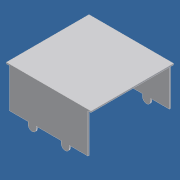
# Autodesk Inventor part: M20_ang_t_shorud2830TX-switch
Saved by Autodesk Inventor 2014 (Build 180170000, 170)
## iProperties
Category: PARTsolutions
Created: 2013-12-29
Part Number: M20_ang_t_shorud2830TX-switch
Catalog Web Link: www.cadenas.de
Description: Angle Mount Miniature Rockers- Switch - Shroud - Series M - Miniature Toggle
Document SubType Name: Modeling
Designer: PARTsolutions
Material: Generic
Density: 1 g/cm^3
Appearance: RGB(192,192,192)
NB: M20_ang_t_shorud2830TX-switch
NN: Angle Mount Miniature Rockers- Switch - Shroud
NT: Series M - Miniature Toggle
NBSYN: $PN.-switch
LINA: M20_ang_t_shorud2830TX-switch
PN: M20_ang_t_shorud2830TX
SRS: M20
PLS: 2
CRCTSALG: '2','2 - ON/NONE/ON','3','3 - ON/OFF/ON','5','5 - ON/NONE/(ON)','8','8 - (ON)/OFF/(ON)','9','9 - ON/OFF/(ON)','4', '4 - ON/ON/ON','6','6 - (ON)/ON/(ON)','7','7 - ON/ON/(ON)'
CRCTS: 8
FRMALG: 'TX', 'TX - Narrow Frame for Small Actuator', 'TZ'  , 'TZ - Wide Frame for Large Actuator'
FRM: TX
TRMNLSALG: '30', '30 - .150" (3.81mm) Right Angle PC (1-3 Pole)', '32'  , '32 -  Right Angle PCB (1 Pole & 0.4VA Rating Only', '40'  , '40 - .150" (3.81mm) Vertical PC (1-4 Pole)', '45'  , '45 - .100" (2.54mm) Vertical PC (1-4 Pole)'
TRMNLS: 30
WIDTH: 0.512
HEIGHT: 0.388
LENGTH: 0.500
A: 0.150
TRMNLNOH: 2.000
TRMNLOV: 3.000
LTRMNL: 0.031
POS: 0.075
POS2: 0.185
POS3: 0.150
D: 0.075
HOLES: 0.185
WH: 0.15000
D1: 0.00000
D2: 0.07500
KT: DUMMY
SUPPLIER: NKKSWITCHES
ARTICLENO: M20_ang_t_shorud2830TX-switch
BOMINFO: M20_ang_t_shorud2830TX-switch
CREATOR: CADENAS GmbH
PSOL_IDENT_0: {$CADENAS_DATA\23d-libs\nkkswitches\toggle\m\parts\m_ang_t_shroud.prj},260 {VTYP=3D},{NB=M20_ang_t_s
PSOL_IDENT_1: horud2830TX-switch},{LINA=M20_ang_t_shorud2830TX-switch},{NN=Angle Mount Miniature Rockers- Switch -
PSOL_IDENT_2: Shroud},{DATE=28.05.2007 07:44:41},{GEOMDATE=28.05.2007 00:00:00},{VERSION=},{LINEID=10},{LINESUBID
PSOL_IDENT_3: =-1},{WBVAR=PLS,CRCTS,FRM,TRMNLS}  {NB=M20_ang_t_shorud2830TX-switch},{LINA=M20_ang_t_shorud2830TX-s
PSOL_IDENT_4: witch},{KT=DUMMY},{PN=M20_ang_t_shorud2830TX},{SRS=M20},{PLS=2},{CRCTSALG='2','2 - ON/NONE/ON','3','
PSOL_IDENT_5: 3 - ON/OFF/ON','5','5 - ON/NONE/(ON)','8','8 - (ON)/OFF/(ON)','9','9 - ON/OFF/(ON)','4', '4 - ON/ON/
PSOL_IDENT_6: ON','6','6 - (ON)/ON/(ON)','7','7 - ON/ON/(ON)'},{CRCTS=8},{FRMALG='TX', 'TX - Narrow Frame for Smal
PSOL_IDENT_7: l Actuator', 'TZ'  , 'TZ - Wide Frame for Large Actuator'},{FRM=TX},{TRMNLSALG='30', '30 - .150\" (3
PSOL_IDENT_8: .81mm) Right Angle PC (1-3 Pole)', '32'  , '32 -  Right Angle PCB (1 Pole & 0.4VA Rating Only', '40'
PSOL_IDENT_9: , '40 - .150\" (3.81mm) Vertical PC (1-4 Pole)', '45'  , '45 - .100\" (2.54mm) Vertical PC (1-4 Po
PSOL_IDENT_10: le)'},{TRMNLS=30},{WIDTH=0.512},{HEIGHT=0.3877},{LENGTH=0.5},{A=0.15},{TRMNLNOH=2},{TRMNLOV=3},{LTRM
PSOL_IDENT_11: NL=0.031},{POS=0.075},{POS2=0.185},{POS3=0.15},{D=0.075},{HOLES=0.185},{WH=0.15000},{D1=0.00000},{D2
PSOL_IDENT_12: =0.07500}
Title: M20_ang_t_shorud2830TX-switch
Author: Cadenas PARTsolutions
Comments: Series M - Miniature Toggle
Autodesk Inventor part; units mm, degrees
sketch "Sketch_1" plane through (0, 0, 0) normal (0, 1, 0) x (-1, 0, 0)
  line L0 (6.5024, 6.35) -> (-6.5024, 6.35)
  line L1 (-6.5024, 6.35) -> (-6.5024, -6.35)
  line L2 (-6.5024, -6.35) -> (6.5024, -6.35)
  line L3 (6.5024, -6.35) -> (6.5024, 6.35)
  constraints: 8 end point
extrude "Extrusion1" add sketch "Sketch_1" along normal blind 0.2032
sketch "Sketch_2" plane through (0, 0, -6.35) normal (0, 0, 1) x (1, 0, 0)
  line L0 (-6.0389, -6.018) -> (-3.1581, -6.018)
  line L1 (-3.1581, -6.018) -> (-3.1581, -6.4159)
  arc A0 (-3.1581, -6.4159) -> (-1.9219, -6.4159) centre (-2.54, -6.4159) ccw
  line L2 (-1.9219, -6.4159) -> (-1.9219, -6.018)
  line L3 (-1.9219, -6.018) -> (1.9219, -6.018)
  line L4 (1.9219, -6.018) -> (1.9219, -6.4159)
  arc A1 (1.9219, -6.4159) -> (3.1581, -6.4159) centre (2.54, -6.4159) ccw
  line L5 (3.1581, -6.4159) -> (3.1581, -6.018)
  line L6 (3.1581, -6.018) -> (6.0389, -6.018)
  line L7 (6.0389, -6.018) -> (6.0389, 0)
  line L8 (6.0389, 0) -> (-6.0389, 0)
  line L9 (-6.0389, 0) -> (-6.0389, -6.018)
  constraints: 20 end point, 4 point on circle, 2 centre point
extrude "Extrusion2" add sketch "Sketch_2" along normal blind 0.2032
sketch "Sketch_3" plane through (0, 0, 6.35) normal (0, 0, 1) x (1, 0, 0)
  line L0 (-6.0389, -6.018) -> (-3.1581, -6.018)
  line L1 (-3.1581, -6.018) -> (-3.1581, -6.4159)
  arc A0 (-3.1581, -6.4159) -> (-1.9219, -6.4159) centre (-2.54, -6.4159) ccw
  line L2 (-1.9219, -6.4159) -> (-1.9219, -6.018)
  line L3 (-1.9219, -6.018) -> (1.9219, -6.018)
  line L4 (1.9219, -6.018) -> (1.9219, -6.4159)
  arc A1 (1.9219, -6.4159) -> (3.1581, -6.4159) centre (2.54, -6.4159) ccw
  line L5 (3.1581, -6.4159) -> (3.1581, -6.018)
  line L6 (3.1581, -6.018) -> (6.0389, -6.018)
  line L7 (6.0389, -6.018) -> (6.0389, 0)
  line L8 (6.0389, 0) -> (-6.0389, 0)
  line L9 (-6.0389, 0) -> (-6.0389, -6.018)
  constraints: 20 end point, 4 point on circle, 2 centre point
extrude "Extrusion3" add sketch "Sketch_3" against normal blind 0.2032
ref_plane "shroud_to_body_XY" through (0, 0, 0) normal (0, 1, 0) x (1, 0, 0)
ref_plane "shroud_to_body_YZ" through (0, 0, 0) normal (1, 0, 0) x (0, 0, -1)
ref_plane "shroud_to_body_ZX" through (0, 0, 0) normal (0, 0, -1) x (0, 1, 0)
body "Solid1"
